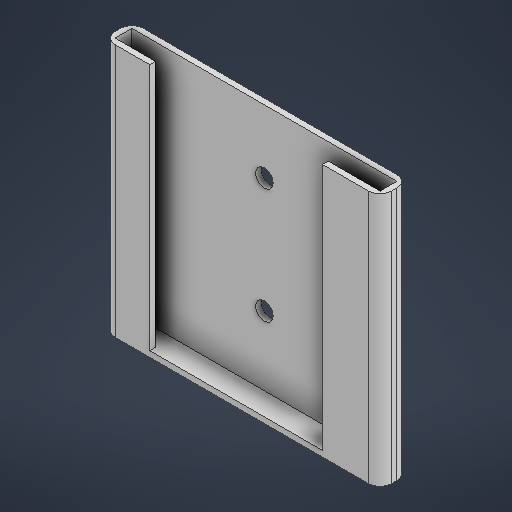
# Autodesk Inventor part: Monitor Seat v1.0
Saved by Autodesk Inventor 2027 (Build 310192060, 192F)
## iProperties
Created: 2026-05-20
Part Number: Monitor Seat v1.0
Material: Generic
Document SubType Name: Modeling
Designer: cheap
Density: 1 g/cm^3
Appearance: Default
Author: cheap
Autodesk Inventor part; units mm, degrees
ref_plane "YZ Plane" through (0, 0, 0) normal (1, 0, 0) x (0, 1, 0)
ref_plane "XZ Plane" through (0, 0, 0) normal (0, 1, 0) x (-1, 0, 0)
ref_plane "XY Plane" through (0, 0, 0) normal (0, 0, 1) x (1, 0, 0)
sketch "Sketch1" plane through (0, 0, 0) normal (0, 1, 0) x (-1, 0, 0)
  line L0 (38.1, 3.9053) -> (-38.1, 3.9052)
  line L1 (-38.1, 3.9052) -> (-38.1, -3.9053)
  line L2 (-38.1, -3.9053) -> (38.1, -3.9052)
  line L3 (38.1, -3.9052) -> (38.1, 3.9053)
  line L4 (38.1, 3.9053) -> (-38.1, -3.9053) construction
  line L5 (-38.1, 3.9052) -> (38.1, -3.9052) construction
  point P0 (0, 0)
  dimension "d0" = 76.2
  dimension "d1" = 7.8105
  constraints: 12 end point, 2 midpoint, 2 parallel, 1 horizontal, 1 perpendicular
  measures "d0" distance of L2.end L1.end
  measures "d1" distance of L1.end L0.end
extrude "Extrusion1" add sketch "Sketch1" along normal blind 1.5875
sketch "Sketch2" plane through (0, 1.5875, 0) normal (0, 1, 0) x (1, 0, 0)
  line L0 (-38.1, -3.9053) -> (38.1, -3.9052) projected
  line L1 (-12.7, -3.9053) -> (-25.4, -3.9053)
  line L2 (-25.4, -3.9053) -> (-25.4, -2.3178)
  line L3 (-38.1, 3.9052) -> (-38.1, -3.9053) projected
  line L4 (-25.4, -2.3178) -> (-36.5125, -2.3178)
  line L5 (-36.5125, -2.3178) -> (-36.5125, 2.3177)
  line L6 (-36.5125, 2.3177) -> (36.5125, 2.3178)
  line L7 (36.5125, 2.3178) -> (36.5125, -2.3177)
  line L8 (36.5125, -2.3177) -> (22.225, -2.3177)
  line L9 (22.225, -2.3177) -> (22.225, -3.9052)
  line L10 (38.1, -3.9052) -> (38.1, 3.9053) projected
  line L11 (38.1, 3.9053) -> (-38.1, 3.9052) projected
  line L12 (-25.4, -3.9053) -> (-38.1, -3.9053)
  line L13 (-38.1, 3.9052) -> (38.1, 3.9053)
  line L14 (38.1, -3.9052) -> (22.225, -3.9052)
  line L15 (38.1, 3.9053) -> (38.1, -3.9052)
  line L16 (-38.1, -3.9053) -> (-38.1, 3.9052)
  point P0 (0, 0)
  dimension "d5" = 12.7
  dimension "d6" = 1.5875
  dimension "d7" = 1.5875
  dimension "d8" = 1.5875
  dimension "d9" = 1.5875
  dimension "d10" = 1.5875
  constraints: 26 end point, 7 perpendicular, 4 collinear, 3 point on line, 1 horizontal
  measures "d5" distance between parallel lines of L3 L2
  measures "d6" distance of L1.end L2.end
  measures "d7" distance of L8.end L9.end
  measures "d8" distance between parallel lines of L10 L7
  measures "d9" distance between parallel lines of L11 L6
  measures "d10" distance between parallel lines of L3 L5
extrude "Extrusion2" add sketch "Sketch2" along normal blind 68.2625 contours L3 L11 L10 L0 L9 L8 L7 L6 L5 L4 L2
sketch "Sketch3" plane through (38.1, 0, -3.9053) normal (0, 0, -1) x (-1, 0, 0)
  circle A0 centre (38.1, 52.3875) radius 2.4343
  circle A1 centre (38.1, 20.6375) radius 2.4343
  line L0 (0, 69.85) -> (76.2, 69.85) projected
  point P0 (38.1, 0)
  point P1 (38.1, 69.85)
  dimension "d13" = 31.75
  dimension "d14" = 17.4625
  constraints: 2 centre point, 1 midpoint
  measures "d13" distance of A1.centre A0.centre
  measures "d14" distance of point (38.1, 69.85) A0.centre
extrude "Extrusion3" cut sketch "Sketch3" against normal blind 68.2625
fillet "Fillet1" radius 3.175 2 edges at (38.1, 34.925, -3.9053) (-38.1, 34.925, -3.9052)
fillet "Fillet2" radius 3.175 2 edges at (-38.1, 34.925, 3.9053) (38.1, 34.925, 3.9052)
body "Solid1"
